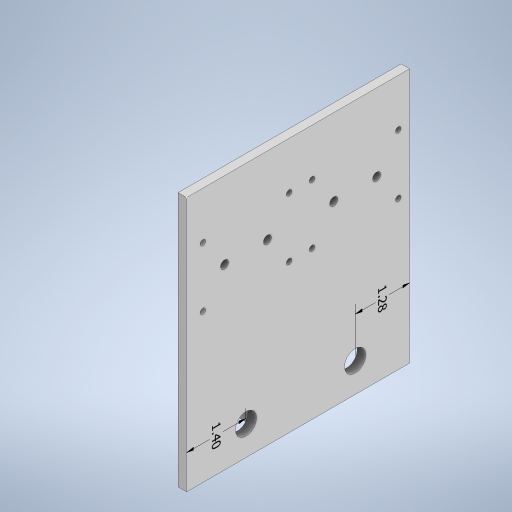
# Autodesk Inventor part: HalfBackWall
Saved by Autodesk Inventor 2024.3 (Build 283343010, 343A)
## iProperties
Created: 2025-04-11
Part Number: HalfBackWall
Material: Generic
Document SubType Name: Modeling
Designer: Vincent Larson
Density: 1 g/cm^3
Appearance: Default
Author: Vincent Larson
Autodesk Inventor part; units mm, degrees
ref_plane "YZ Plane" through (0, 0, 0) normal (1, 0, 0) x (0, 1, 0)
ref_plane "XZ Plane" through (0, 0, 0) normal (0, 1, 0) x (-1, 0, 0)
ref_plane "XY Plane" through (0, 0, 0) normal (0, 0, 1) x (1, 0, 0)
sketch "Sketch4" plane through (0, 0, 0) normal (1, 0, 0) x (0, 1, 0)
  line L0 (0, 0) -> (-152.4, 0)
  line L1 (-152.4, 0) -> (-152.4, -133.35)
  line L2 (-152.4, -133.35) -> (0, -133.35)
  line L3 (0, -133.35) -> (0, 0)
  dimension "d10" = 152.4
  dimension "d11" = 133.35
  constraints: 8 end point, 2 parallel, 1 horizontal, 1 perpendicular
  measures "d10" distance of L2.end L1.end
  measures "d11" distance of L1.end L0.end
extrude "Extrusion2" add sketch "Sketch4" along normal blind 5.08
sketch "Sketch5" plane through (5.08, 0, 0) normal (1, 0, 0) x (0, 0, -1)
  line L0 (133.35, 0) -> (0, 0) projected
  line L1 (66.675, 0) -> (66.675, -152.4)
  line L2 (0, -152.4) -> (133.35, -152.4) projected
  circle A0 centre (126.5334, -28.194) radius 1.651
  circle A1 centre (74.9714, -28.194) radius 1.651
  circle A2 centre (61.2554, -28.194) radius 1.651
  circle A3 centre (9.6934, -28.194) radius 1.651
  circle A4 centre (126.5334, -63.754) radius 1.651
  circle A5 centre (74.9714, -63.754) radius 1.651
  circle A6 centre (61.2554, -63.754) radius 1.651
  circle A7 centre (9.6934, -63.754) radius 1.651
  circle A8 centre (113.5794, -45.974) radius 2.413
  circle A9 centre (87.9254, -45.974) radius 2.413
  circle A10 centre (48.3014, -45.974) radius 2.413
  circle A11 centre (22.6474, -45.974) radius 2.413
  line L3 (66.675, 0) -> (66.675, -28.194)
  line L4 (66.675, -28.194) -> (73.533, -28.194)
  line L5 (73.533, -28.194) -> (66.675, -28.194)
  line L6 (66.675, -28.194) -> (59.817, -28.194)
  dimension "d14" = 28.194
  dimension "d15" = 6.858
  dimension "d16" = 6.858
  constraints: 12 centre point, 10 end point, 2 midpoint, 2 point on line, 1 collinear, 1 horizontal
  measures "d14" distance of L1.start L3.end
  measures "d15" distance of L3.end L4.end
  measures "d16" distance of L3.end L6.end
extrude "Extrusion3" cut sketch "Sketch5" against normal blind 5.08
sketch "Sketch6" plane through (5.08, 0, 0) normal (1, 0, 0) x (0, 0, -1)
  circle A0 centre (22.6474, -45.974) radius 2.413 projected
  circle A1 centre (48.3014, -45.974) radius 2.413 projected
  line L0 (0, -152.4) -> (133.35, -152.4) projected
  circle A2 centre (35.4744, -134.874) radius 6.35
  circle A3 centre (87.9254, -45.974) radius 2.413 projected
  circle A4 centre (113.5794, -45.974) radius 2.413 projected
  circle A5 centre (100.7524, -134.874) radius 6.35
  point P0 (0, 0)
  dimension "d20" = 12.7
  dimension "d22" = 12.7
  constraints: 2 centre point
  measures "d20" diameter of A2
  measures "d22" diameter of A5
extrude "Extrusion4" cut sketch "Sketch6" against normal blind 5.08 contours A2 | A5
sketch "Sketch7" plane through (0, 0, 0) normal (-1, 0, 0) x (0, 0, 1)
  line L0 (-133.35, 0) -> (0, 0) projected
  line L1 (-66.675, 0) -> (-66.675, -152.4)
  line L2 (0, -152.4) -> (-133.35, -152.4) projected
  line L3 (-79.375, -107.9503) -> (-53.975, -107.9503)
  line L4 (-53.975, -107.9503) -> (-53.975, -152.4)
  line L5 (-53.975, -152.4) -> (-79.375, -152.4)
  line L6 (-79.375, -152.4) -> (-79.375, -107.9503)
  line L7 (-79.375, -107.9503) -> (-53.975, -152.4) construction
  line L8 (-53.975, -107.9503) -> (-79.375, -152.4) construction
  point P0 (-66.675, -130.1752)
  dimension "d29" = 25.4
  constraints: 14 end point, 4 midpoint, 2 parallel, 2 point on line, 1 horizontal, 1 perpendicular
  measures "d29" distance of L4.end L5.end
extrude "Extrusion5" add sketch "Sketch7" along normal blind 25.4
sketch "Sketch8" plane through (0, -152.4, -79.375) normal (0, 0, -1) x (-1, 0, 0)
  line L0 (25.4, 0) -> (25.4, 44.4497) projected
  line L1 (0, 44.4497) -> (25.4, 44.4497) projected
  line L2 (25.4, 0) -> (0, 44.4497)
  point P0 (0, 152.4)
  constraints: 2 end point
extrude "Extrusion6" cut sketch "Sketch8" against normal blind 25.4
sketch "Sketch9" plane through (5.08, 0, 0) normal (1, 0, 0) x (0, 0, -1)
  point P0 (0, 0)
body "Solid2"
